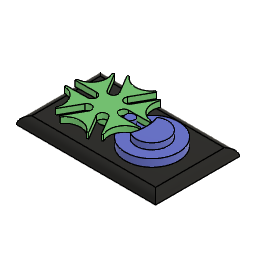
2nd_mechanism (Autodesk Fusion 360 design; units mm, degrees)
Autodesk Fusion 360 part; units mm, degrees
sketch "HolderSketch" plane through (0, 0, 0) normal (0, 0, 1) x (1, 0, 0) in component "Holder"
  circle A0 centre (65, 55) radius 10
  line L0 (0, 0) -> (182.5, 0)
  line L1 (182.5, 0) -> (182.5, 110)
  line L2 (182.5, 110) -> (0, 110)
  line L3 (0, 110) -> (0, 0)
  dimension "d2" = 182.5
  dimension "d3" = 110
  constraint horizontal L0
  constraint vertical L1
  constraint horizontal L2
  constraint vertical L3
  constraint coincident L0.start L3.end
  measures "d2" distance of L0.start L0.end
  measures "d3" distance of L0.start L2.end
extrude "Extrude1" add sketch "HolderSketch" along normal blind 10 contours A0 | L0 L1 L2 L3 makes body 1 in component "Holder"
extrude "Extrude2" add sketch "HolderSketch" along normal blind 20 contours A0 bodies 1 in component "Holder"
fillet "Fillet1" radius 10 4 edges at (91.25, 0, 10) (0, 55, 10) (91.25, 110, 10) (182.5, 55, 10) on bodies 1 in component "Holder"
sketch "CrankSketch" plane through (0, 0, 10) normal (0, 0, 1) x (-1, 0, 0) in component "Crank"
  circle A0 centre (-122.735, -55) radius 34.8501
  arc A1 (-111.7948, -37.3861) -> (-111.7948, -72.614) centre (-122.735, -55) ccw
  arc A2 (-111.7948, -37.3861) -> (-111.7948, -72.614) centre (-65, -55) ccw
  circle A3 centre (-93.8691, -55.3464) radius 5.991
  dimension "d57" = 28.868
  dimension "d58" = 11.982
  measures "d57" distance of A0.centre A3.centre
  measures "d58" diameter of A3
extrude "Extrude3" add sketch "CrankSketch" along normal blind 9.8 separate body contours A0 A3 | A0 A3 | A1 A2 picked at (-100.8665, -40.9991) picked at (-95.8515, -55.6544) makes body 2 in component "Crank"
extrude "Extrude4" add sketch "CrankSketch" along normal blind 17.8 contours A0 A3 | A1 A2 picked at (-95.8515, -55.6544) bodies 2 in component "Crank"
sketch "WheelSketch" plane through (0, 0, 20) normal (0, 0, 1) x (-1, 0, 0) in component "Wheel"
  circle A0 centre (-65, -55) radius 10
  arc A1 (-110.9374, -72.0516) -> (-110.9374, -37.9484) centre (-122.735, -55) ccw
  circle A2 centre (-65, -55) radius 10
  arc A3 (-73.2016, -103.3087) -> (-102.7358, -86.2572) centre (-93.8675, -105) ccw
  arc A4 (-27.2642, -86.2571) -> (-56.7984, -103.3087) centre (-36.1325, -105) ccw
  arc A5 (-19.0626, -37.9484) -> (-19.0626, -72.0516) centre (-7.265, -55) ccw
  arc A6 (-56.7984, -6.6913) -> (-27.2642, -23.7428) centre (-36.1325, -5) ccw
  arc A7 (-102.7358, -23.7429) -> (-73.2016, -6.6913) centre (-93.8675, -5) ccw
  circle A8 centre (-65, -55) radius 12
  line L0 (-104.1159, -84.5117) -> (-79.7577, -70.4485)
  line L1 (-110.1159, -74.1194) -> (-85.7576, -60.0562)
  line L2 (-104.9338, -84.984) -> (-104.9884, -85.0155)
  arc A9 (-79.7577, -70.4485) -> (-85.7576, -60.0562) centre (-82.7576, -65.2524) ccw
  line L3 (-59, -103.6313) -> (-59, -75.5048)
  line L4 (-71, -103.6313) -> (-71, -75.5047)
  arc A10 (-59, -75.5048) -> (-71, -75.5047) centre (-65, -75.5048) ccw
  line L5 (-19.8841, -74.1195) -> (-44.2424, -60.0562)
  line L6 (-25.8841, -84.5118) -> (-50.2424, -70.4485)
  arc A11 (-44.2424, -60.0562) -> (-50.2424, -70.4485) centre (-47.2424, -65.2524) ccw
  line L7 (-25.8841, -25.4883) -> (-50.2423, -39.5515)
  line L8 (-19.8841, -35.8806) -> (-44.2424, -49.9438)
  arc A12 (-50.2423, -39.5515) -> (-44.2424, -49.9438) centre (-47.2424, -44.7476) ccw
  line L9 (-71, -6.3687) -> (-71, -34.4952)
  line L10 (-59, -6.3687) -> (-59, -34.4953)
  arc A13 (-71, -34.4952) -> (-59, -34.4953) centre (-65, -34.4952) ccw
  line L11 (-110.1159, -35.8805) -> (-85.7576, -49.9438)
  line L12 (-104.1159, -25.4882) -> (-79.7576, -39.5515)
  arc A14 (-85.7576, -49.9438) -> (-79.7576, -39.5515) centre (-82.7576, -44.7476) ccw
  arc A15 (-56.7984, -6.6913) -> (-59, -6.3687) centre (-65, -55) ccw
  arc A16 (-71, -6.3687) -> (-73.2016, -6.6913) centre (-65, -55) ccw
  arc A17 (-102.7358, -23.7429) -> (-104.1159, -25.4882) centre (-65, -55) ccw
  arc A18 (-110.1159, -35.8805) -> (-110.9374, -37.9484) centre (-65, -55) ccw
  arc A19 (-110.9374, -72.0516) -> (-110.1159, -74.1194) centre (-65, -55) ccw
  arc A20 (-104.1159, -84.5117) -> (-102.7358, -86.2572) centre (-65, -55) ccw
  arc A21 (-73.2016, -103.3087) -> (-71, -103.6313) centre (-65, -55) ccw
  arc A22 (-59, -103.6313) -> (-56.7984, -103.3087) centre (-65, -55) ccw
  arc A23 (-27.2642, -86.2571) -> (-25.8841, -84.5118) centre (-65, -55) ccw
  arc A24 (-19.8841, -74.1195) -> (-19.0626, -72.0516) centre (-65, -55) ccw
  arc A25 (-19.0626, -37.9484) -> (-19.8841, -35.8806) centre (-65, -55) ccw
  arc A26 (-25.8841, -25.4883) -> (-27.2642, -23.7428) centre (-65, -55) ccw
  dimension "d74" = 2
  dimension "d88" = 12
  dimension "d95" = 98
  constraint parallel L0 L2
  constraint coincident A6.start A16
  constraint concentric A15 A16
  constraint concentric A16 A17
  constraint concentric A17 A18
  constraint concentric A18 A19
  constraint concentric A19 A20
  constraint concentric A20 A21
  constraint concentric A21 A22
  constraint concentric A22 A23
  constraint concentric A23 A24
  constraint concentric A24 A25
  constraint concentric A25 A26
  measures "d88" diameter of A9
  measures "d95" diameter of A16
extrude "Extrude1'" add sketch "WheelSketch" along normal blind 1 and the other way blind 8 separate body contours A8 makes body 3 in component "Wheel"
extrude "Extrude2'" add sketch "WheelSketch" along normal blind 7.5 from surface at 1 contours A0 A2 | A1 A3 A4 A5 A6 A7 L0 L1 A9 L3 L4 A10 L5 L6 A11 L7 L8 A12 L9 L10 A13 L11 L12 A14 A15 A16 A17 A18 A19 A20 A21 A22 A23 A24 A25 A26 | A8 bodies 3 in component "Wheel"
component "Holder" placed x (1, 0, 0) y (0, 1, 0) z (0, 0, 1) at (0, 0, 0)
component "Crank" placed x (1, 0, 0) y (0, 1, 0) z (0, 0, 1) at (0, 0, 0)
component "Wheel" placed x (-0.872115, 0.489302, 0) y (-0.489302, -0.872115, 0) z (0, 0, 1) at (148.599, 71.1617, 0)
equation "d61 = 8 mm + 9.8 mm"
named bodies: "HolderBody", "CrankBody", "WheelBody"
